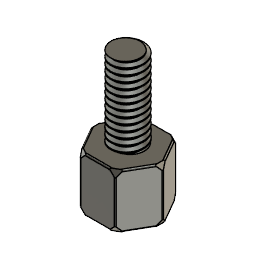
M2.5 X 4mm Male to Female Standoff (Autodesk Fusion 360 design; units mm, degrees)
Autodesk Fusion 360 part; units mm, degrees
sketch "Sketch1" plane through (0, 0, 0) normal (0, 0, 1) x (1, 0, 0)
  circle A0 centre (0, 0) radius 1.25
  line L0 (2.6, 0) -> (1.3, 2.2517)
  line L1 (1.3, 2.2517) -> (-1.3, 2.2517)
  line L2 (-1.3, 2.2517) -> (-2.6, 0)
  line L3 (-2.6, 0) -> (-1.3, -2.2517)
  line L4 (-1.3, -2.2517) -> (1.3, -2.2517)
  line L5 (1.3, -2.2517) -> (2.6, 0)
  circle A1 centre (0, 0) radius 2.2517
  dimension "d1" = 2.5
  dimension "d2" = 2.6
  constraint coincident A0.centre A1.centre
  constraint concentric A0 A1
  constraint tangent L0 A1
  measures "d1" diameter of A0
  measures "d2" distance of L0.start A0.centre
extrude "Extrude1" add sketch "Sketch1" along normal blind 4 contours A0 | L0 L5 A1 | L0 L1 A1 | A1 | L4 L5 A1 | L1 L2 A1 | L3 L4 A1 | L2 L3 A1
extrude "Extrude2" cut sketch "Sketch1" along normal blind 3 contours A0
extrude "Extrude3" add sketch "Sketch1" along normal blind 6 from surface at 4 contours A0
thread "Thread1" "ISO Metric profile 2.5 M2.5x0.45 M2.5x0.45 6H" major diameter 2.58 minor diameter 2.0755 pitch 0.45 angle 60 modelled right hand crest width 0.1211 on face at (1.2484, -0.0623, 2) crest through (1.0377, 0, 0.1125)
thread "Thread2" "ISO Metric profile 2.5 M2.5x0.45 M2.5x0.45 6g" major diameter 2.43 minor diameter 1.9165 pitch 0.45 angle 60 modelled right hand crest width 0.0648 on face at (1.2484, 0.0623, 6) crest through (1.215, 0, 3.8875)
sketch "Sketch2" plane through (0, 0, 0) normal (0, 0, -1) x (1, 0, 0)
  spline S0 degree 3 poles (-0.3352, -1.2457) (-0.4889, -1.188) (-0.6302, -1.1014) (-0.8662, -0.8823) (-0.9603, -0.7537) (-1.0902, -0.4727) (-1.1269, -0.3241) (-1.1397, -0.0273) (-1.1182, 0.1179) (-1.0385, 0.3388) (-0.9979, 0.4189) (-0.8989, 0.565) (-0.8414, 0.6308) (-0.7764, 0.6886) knots 0 0 0 0 0.049266 0.049266 0.096695 0.096695 0.142284 0.142284 0.186034 0.186034 0.212977 0.212977 0.239179 0.239179 0.239179 0.239179
  arc A0 (0.7764, 0.6886) -> (-0.7764, 0.6886) centre (0, 0) ccw
  spline S1 degree 3 poles (0.7764, 0.6886) (0.879, 0.5975) (0.9623, 0.4868) (1.0858, 0.2347) (1.1226, 0.0946) (1.1419, -0.198) (1.122, -0.3478) (1.0249, -0.6378) (0.9464, -0.7743) (0.7769, -0.9706) (0.6998, -1.0398) (0.5283, -1.1593) (0.4342, -1.2086) (0.3352, -1.2457) knots 0 0 0 0 0.041153 0.041153 0.08414 0.08414 0.128959 0.128959 0.17561 0.17561 0.20647 0.20647 0.238077 0.238077 0.238077 0.238077
  arc A1 (-0.3352, -1.2457) -> (0.3352, -1.2457) centre (0, 0) ccw
  line L0 (2.6, 0) -> (1.3, 2.2517)
  line L1 (1.3, 2.2517) -> (-1.3, 2.2517)
  line L2 (-1.3, 2.2517) -> (-2.6, 0)
  line L3 (-2.6, 0) -> (-1.3, -2.2517)
  line L4 (-1.3, -2.2517) -> (1.3, -2.2517)
  line L5 (1.3, -2.2517) -> (2.6, 0)
  line L6 (-2.6, 0) -> (-2.475, -0.2165)
  line L7 (-2.6, 0) -> (-2.475, 0.2165)
  dimension "d14" = 0.25
  dimension "d15" = 0.25
  constraint coincident L2.end L3.start
  constraint parallel L3 L6
  constraint parallel L2 L7
  measures "d14" distance of L2.end L6.end
  measures "d15" distance of L2.end L7.end
ref_plane "WorkPlane1" through (-2.6, 0, 0) normal (1, 0, 0) x (0, 1, 0)
sketch "Sketch3" plane through (-2.6, 0, 0) normal (1, 0, 0) x (0, 1, 0)
  line L0 (0, 0) -> (0, 0.25)
  line L1 (0, 4) -> (0, 3.75)
  dimension "d17" = 0.25
  dimension "d23" = 0.25
  constraint coincident L0.start origin
  constraint vertical L0
  constraint vertical L1
  measures "d17" distance of L0.start L0.end
  measures "d23" distance of L1.start L1.end
ref_plane "WorkPlane2" through (-2.6, 0, 0.25) normal (-0.894427, 0, -0.447214) x (-0.447214, 0, 0.894427)
sketch "Sketch4" plane through (-1.98, 0, -0.99) normal (-0.894427, 0, -0.447214) x (-0.447214, 0, 0.894427)
  line L0 (1.45, -0.25) -> (1, -0.25)
  line L1 (1, -0.25) -> (1, 0.25)
  line L2 (1, 0.25) -> (1.45, 0.25)
  line L3 (1.45, 0.25) -> (1.45, -0.25)
  constraint horizontal L0
  constraint vertical L1
  constraint horizontal L2
  constraint vertical L3
extrude "Extrude4" cut sketch "Sketch4" along normal blind 5
move_face "OffsetFaces1" offset -0.1 1 faces at (-2.5167, 0, 0.0833)
pattern_circular "C-Pattern1" count 6 over 360 about axis through (0, 0, 1.75) along (0, 0, 1) of 1 faces at (-2.4421, 0, 0.1579)
sketch "Sketch5" plane through (0, 0, 4) normal (0, 0, 1) x (-1, 0, 0)
  arc A0 (-0.531, -1.0928) -> (0.531, -1.0928) centre (0, 0) ccw
  spline S0 degree 3 poles (-0.531, -1.0928) (-0.6224, -1.0363) (-0.7058, -0.9678) (-0.8498, -0.8123) (-0.9102, -0.7265) (-1.025, -0.5043) (-1.0664, -0.3633) (-1.0913, -0.0796) (-1.0769, 0.0603) (-0.9959, 0.3203) (-0.9325, 0.4387) (-0.7669, 0.6389) (-0.6682, 0.7204) (-0.5564, 0.7801) knots -0.22638 -0.22638 -0.22638 -0.22638 -0.19429 -0.19429 -0.163068 -0.163068 -0.119555 -0.119555 -0.077873 -0.077873 -0.038021 -0.038021 0 0 0 0
  arc A1 (0.5564, 0.7801) -> (-0.5564, 0.7801) centre (0, 0) ccw
  spline S1 degree 3 poles (0.5564, 0.7801) (0.6331, 0.7392) (0.7038, 0.6879) (0.8319, 0.5661) (0.8882, 0.4956) (1.0044, 0.3025) (1.0504, 0.1735) (1.0924, -0.1007) (1.0857, -0.2438) (1.0175, -0.5256) (0.9543, -0.6611) (0.7768, -0.9059) (0.6623, -1.0116) (0.531, -1.0928) knots -0.227524 -0.227524 -0.227524 -0.227524 -0.201332 -0.201332 -0.17428 -0.17428 -0.133466 -0.133466 -0.090815 -0.090815 -0.046326 -0.046326 0 0 0 0
  line L0 (-1.3, 2.2517) -> (-2.6, 0)
  line L1 (-2.6, 0) -> (-1.3, -2.2517)
  line L2 (-1.3, -2.2517) -> (1.3, -2.2517)
  line L3 (1.3, -2.2517) -> (2.6, 0)
  line L4 (2.6, 0) -> (1.3, 2.2517)
  line L5 (1.3, 2.2517) -> (-1.3, 2.2517)
  line L6 (2.6, 0) -> (2.475, 0.2165)
  line L7 (2.6, 0) -> (2.475, -0.2165)
  dimension "d24" = 0.25
  dimension "d25" = 0.25
  constraint coincident L3.end L4.start
  constraint parallel L4 L6
  constraint parallel L3 L7
  measures "d24" distance of L3.end L6.end
  measures "d25" distance of L3.end L7.end
ref_plane "WorkPlane3" through (-2.475, 0.2165, 4) normal (0.894427, 0, -0.447213) x (-0.447213, 0, -0.894427)
sketch "Sketch6" plane through (-3.58, 0, 1.79) normal (0.894427, 0, -0.447213) x (-0.447213, 0, -0.894427)
  line L0 (-2.7, 0.3) -> (-2.1, 0.3)
  line L1 (-2.1, 0.3) -> (-2.1, -0.3)
  line L2 (-2.1, -0.3) -> (-2.7, -0.3)
  line L3 (-2.7, -0.3) -> (-2.7, 0.3)
  constraint horizontal L0
  constraint vertical L1
  constraint horizontal L2
  constraint vertical L3
extrude "Extrude5" cut sketch "Sketch6" against normal blind 4
move_face "OffsetFaces2" offset -0.1 1 faces at (-2.5167, 0, 3.9167)
pattern_circular "C-Pattern2" count 6 over 360 about axis through (0, 0, 1.75) along (0, 0, 1) of 1 faces at (-2.4421, 0, 3.8421)
fillet "Fillet1" radius 0.1 18 edges at (-1.3, 2.2517, 2) (-2.6, 0, 2) (-1.3, -2.2517, 2) (1.3, -2.2517, 2) (2.6, 0, 2) (1.3, 2.2517, 2) (0, 2.2517, 4) (1.95, 1.1258, 4) (1.95, -1.1258, 4) (0, -2.2517, 4) (-1.95, -1.1258, 4) (-1.95, 1.1258, 4) (-1.95, -1.1258, 0) (-1.95, 1.1258, 0) (0, 2.2517, 0) (1.95, 1.1258, 0) (1.95, -1.1258, 0) (0, -2.2517, 0)
